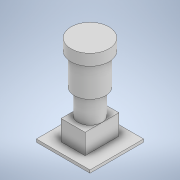
# Autodesk Inventor part: Camera
Saved by Autodesk Inventor 2020 (Build 240168000, 168)
## iProperties
Created: 2019-07-19
Part Number: Camera
Material: Generic
Document SubType Name: Modeling
Designer: Paul
Density: 1 g/cm^3
Appearance: Default
Author: Paul
Autodesk Inventor part; units mm, degrees
ref_plane "YZ Plane" through (0, 0, 0) normal (1, 0, 0) x (0, 1, 0)
ref_plane "XZ Plane" through (0, 0, 0) normal (0, 1, 0) x (-1, 0, 0)
ref_plane "XY Plane" through (0, 0, 0) normal (0, 0, 1) x (1, 0, 0)
sketch "Sketch1" plane through (0, 0, 0) normal (0, 1, 0) x (-1, 0, 0)
  line L0 (19, 19) -> (-19, 19)
  line L1 (-19, 19) -> (-19, -19)
  line L2 (-19, -19) -> (19, -19)
  line L3 (19, -19) -> (19, 19)
  line L4 (19, 19) -> (-19, -19) construction
  line L5 (-19, 19) -> (19, -19) construction
  point P0 (0, 0)
  dimension "d0" = 38
  dimension "d1" = 38
  constraints: 12 end point, 2 midpoint, 2 parallel, 1 horizontal, 1 perpendicular
  measures "d0" distance of L2.end L1.end
  measures "d1" distance of L1.end L0.end
extrude "Extrusion1" add sketch "Sketch1" along normal blind 2
sketch "Sketch2" plane through (0, 2, 0) normal (0, 1, 0) x (1, 0, 0)
  line L0 (8.5, -12) -> (-8.5, -12)
  line L1 (-8.5, -12) -> (-8.5, 12)
  line L2 (-8.5, 12) -> (8.5, 12)
  line L3 (8.5, 12) -> (8.5, -12)
  line L4 (8.5, -12) -> (-8.5, 12) construction
  line L5 (-8.5, -12) -> (8.5, 12) construction
  point P0 (0, 0)
  dimension "d4" = 17
  dimension "d5" = 24
  constraints: 12 end point, 2 midpoint, 2 parallel, 1 horizontal, 1 perpendicular
  measures "d4" distance of L1.end L2.end
  measures "d5" distance of L0.end L1.end
extrude "Extrusion2" add sketch "Sketch2" along normal blind 14.34
sketch "Sketch3" plane through (0, 16.34, 0) normal (0, 1, 0) x (1, 0, 0)
  circle A0 centre (0, 0) radius 8.45
  dimension "d8" = 16.9
  constraints: 1 centre point, 1 coincident
  measures "d8" diameter of A0
extrude "Extrusion3" add sketch "Sketch3" along normal blind 17.7
sketch "Sketch4" plane through (0, 34.04, 0) normal (0, 1, 0) x (1, 0, 0)
  circle A0 centre (0, 0) radius 11
  dimension "d13" = 22
  constraints: 1 centre point, 1 coincident
  measures "d13" diameter of A0
extrude "Extrusion4" add sketch "Sketch4" along normal blind 22
sketch "Sketch5" plane through (0, 56.04, 0) normal (0, 1, 0) x (1, 0, 0)
  circle A0 centre (0, 0) radius 13.45
  dimension "d16" = 26.9
  constraints: 1 centre point, 1 coincident
  measures "d16" diameter of A0
extrude "Extrusion5" add sketch "Sketch5" along normal blind 8
body "Solid1"
